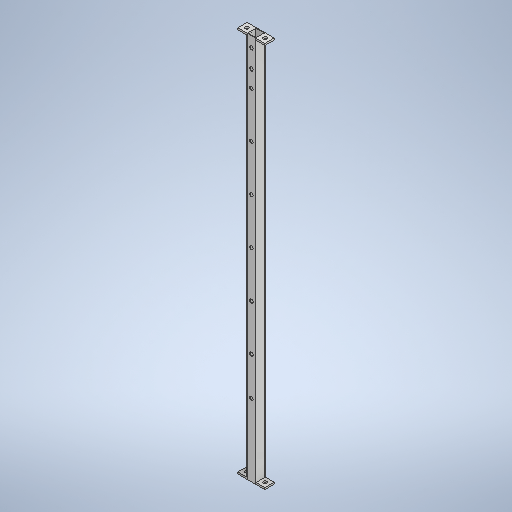
# Autodesk Inventor part: Perfil_Vertical_Acero
Saved by Autodesk Inventor 2025.2 (Build 292293000, 293)
## iProperties
Created: 2025-05-30
Part Number: Perfil_Vertical_Acero
Material: Generic
Document SubType Name: Modeling
Designer: USER
Density: 1 g/cm^3
Appearance: Default
Author: USER
Autodesk Inventor part; units mm, degrees
ref_plane "YZ Plane" through (0, 0, 0) normal (1, 0, 0) x (0, 1, 0)
ref_plane "XZ Plane" through (0, 0, 0) normal (0, 1, 0) x (-1, 0, 0)
ref_plane "XY Plane" through (0, 0, 0) normal (0, 0, 1) x (1, 0, 0)
sketch "Sketch1" plane through (0, 0, 0) normal (0, 1, 0) x (-1, 0, 0)
  line L0 (0, 0) -> (31.75, 0)
  line L1 (31.75, 0) -> (31.75, -31.75)
  line L2 (31.75, -31.75) -> (0, -31.75)
  line L3 (0, -31.75) -> (0, 0)
  line L4 (29.75, -29.75) -> (29.75, -2)
  line L5 (29.75, -2) -> (2, -2)
  line L6 (2, -2) -> (2, -29.75)
  line L7 (2, -29.75) -> (29.75, -29.75)
  dimension "d8" = 31.75
  dimension "d9" = 31.75
  dimension "d10" = 2
  constraints: 16 end point, 4 parallel, 2 perpendicular, 1 horizontal, 3 other
  measures "d8" distance of L0.end L1.end
  measures "d9" distance of L1.end L2.end
  measures "d10" distance between parallel lines of L1 L4
extrude "Extrusion1" add sketch "Sketch1" along normal blind 1310
sketch "Sketch3" plane through (-31.75, 0, 0) normal (0, 0, 1) x (1, 0, 0)
  line L0 (31.75, 0) -> (31.75, 368)
  line L1 (31.75, 0) -> (31.75, 1310) projected
  line L2 (0, 0) -> (31.75, 0) projected
  line L3 (31.75, 0) -> (31.75, 1310) projected
  line L4 (0, 1310) -> (31.75, 1310) projected
  line L5 (0, 0) -> (0, 1310) projected
  circle A0 centre (15.875, 375) radius 6
  circle A1 centre (15.875, 531) radius 6
  circle A2 centre (15.875, 687) radius 6
  circle A3 centre (15.875, 843) radius 6
  circle A4 centre (15.875, 999) radius 6
  circle A5 centre (15.875, 1155) radius 6
  dimension "d11" = 368
  dimension "d12" = 12
  dimension "d15" = 12
  dimension "d16" = 156
  dimension "d17" = 12
  dimension "d18" = 156
  dimension "d19" = 12
  dimension "d20" = 156
  dimension "d21" = 12
  dimension "d22" = 156
  dimension "d23" = 12
  dimension "d24" = 156
  constraints: 6 centre point, 2 end point, 1 point on line
  measures "d11" distance of L0.start L0.end
  measures "d12" diameter of A0
  measures "d15" diameter of A1
  measures "d16" distance of A0.centre A1.centre
  measures "d17" diameter of A2
  measures "d18" distance of A2.centre A1.centre
  measures "d19" diameter of A3
  measures "d20" distance of A2.centre A3.centre
  measures "d21" diameter of A4
  measures "d22" distance of A4.centre A3.centre
  measures "d23" diameter of A5
  measures "d24" distance of A4.centre A5.centre
extrude "Extrusion2" cut sketch "Sketch3" against normal through all contours A0 | A1 | A2 | A3 | A4 | A5
sketch "Sketch4" plane through (0, 0, 0) normal (0, -1, 0) x (1, 0, 0)
  line L0 (0, -31.75) -> (-31.75, -31.75) projected
  line L1 (0, 0) -> (0, -31.75) projected
  line L2 (-31.75, 0) -> (0, 0) projected
  line L3 (-31.75, -31.75) -> (-31.75, 0) projected
  line L4 (-29.75, -29.75) -> (-2, -29.75) projected
  line L5 (-29.75, -2) -> (-29.75, -29.75) projected
  line L6 (-2, -2) -> (-29.75, -2) projected
  line L7 (-2, -29.75) -> (-2, -2) projected
  line L8 (0, 0) -> (30, 0)
  line L9 (30, 0) -> (30, -31.75)
  line L10 (30, -31.75) -> (0, -31.75)
  line L11 (0, -31.75) -> (0, 0)
  line L12 (-31.75, 0) -> (-61.75, 0)
  line L13 (-61.75, 0) -> (-61.75, -31.75)
  line L14 (-61.75, -31.75) -> (-31.75, -31.75)
  line L15 (-31.75, -31.75) -> (-31.75, 0)
  circle A0 centre (-46.75, -15.875) radius 6
  circle A1 centre (15, -15.875) radius 6
  dimension "d25" = 30
  dimension "d26" = 30
  dimension "d29" = 12
  dimension "d30" = 12
  constraints: 16 end point, 4 parallel, 2 centre point, 2 horizontal, 2 perpendicular, 1 point on line
  measures "d25" distance of L9.end L10.end
  measures "d26" distance of L14.end L13.end
  measures "d29" diameter of A0
  measures "d30" diameter of A1
extrude "Extrusion3" add sketch "Sketch4" against normal blind 6 contours L1 L8 L9 L10 | L14 L13 L12 L3
sketch "Sketch5" plane through (0, 1310, 0) normal (0, 1, 0) x (1, 0, 0)
  line L0 (0, 31.75) -> (-31.75, 31.75) projected
  line L1 (30, 0) -> (-61.75, 0) projected
  line L2 (0, 31.75) -> (30, 31.75)
  line L3 (30, 31.75) -> (30, 0)
  line L4 (30, 0) -> (0, 0)
  line L5 (0, 0) -> (0, 31.75)
  line L6 (-31.75, 31.75) -> (-31.75, 0) projected
  line L7 (-61.75, 31.75) -> (-61.75, 0) projected
  line L8 (-31.75, 31.75) -> (-61.75, 31.75)
  line L9 (-61.75, 31.75) -> (-61.75, 0)
  line L10 (-61.75, 0) -> (-31.75, 0)
  line L11 (-31.75, 0) -> (-31.75, 31.75)
  circle A0 centre (-46.75, 15.875) radius 6 projected
  circle A1 centre (-46.75, 15.875) radius 6
  circle A2 centre (15, 15.875) radius 6 projected
  circle A3 centre (15, 15.875) radius 6
  constraints: 16 end point, 4 parallel, 2 centre point, 2 coincident, 2 horizontal, 2 perpendicular
extrude "Extrusion4" add sketch "Sketch5" against normal blind 6 contours L2 L3 L1 L5 | L6 L1 L7 L8
sketch "Sketch6" plane through (-61.75, 0, 0) normal (0, 0, 1) x (1, 0, 0)
  circle A0 centre (45.875, 1274) radius 6
  line L0 (91.75, 1304) -> (61.75, 1304) projected
  circle A1 centre (45.875, 1212.25) radius 6
  point P0 (61.75, 0)
  dimension "d33" = 12
  dimension "d34" = 30
  dimension "d35" = 12
  dimension "d36" = 61.75
  constraints: 2 centre point
  measures "d33" diameter of A0
  measures "d34" distance from line of L0 A0.centre
  measures "d35" diameter of A1
  measures "d36" distance of A1.centre A0.centre
extrude "Extrusion5" cut sketch "Sketch6" against normal through all
sketch "Sketch7" plane through (-61.75, 0, 0) normal (0, 0, 1) x (1, 0, 0)
  circle A0 centre (45.875, 245) radius 6
  circle A1 centre (45.875, 375) radius 6 projected
  point P0 (61.75, 0)
  dimension "d39" = 12
  dimension "d40" = 130
  constraints: 1 centre point
  measures "d39" diameter of A0
  measures "d40" distance of A0.centre A1.centre
extrude "Extrusion6" cut sketch "Sketch7" against normal through all contours A0
body "Solid1"
